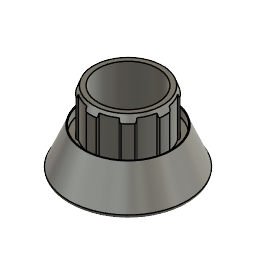
Fuß Tisch Keller (Autodesk Fusion 360 design; units mm, degrees)
Autodesk Fusion 360 part; units mm, degrees
sketch "Skizze1" plane through (0, 0, 0) normal (1, 0, 0) x (0, 0, -1)
  line L0 (0, 0) -> (-24, 0)
  line L1 (-24.9209, 1.3899) -> (-18.1, 17.5)
  line L2 (-18.1, 17.5) -> (-18.1, 13)
  line L3 (-18.1, 13) -> (-15, 13)
  line L4 (-15, 13) -> (-15, 31)
  line L5 (-15, 31) -> (-12.5, 31)
  line L6 (-12.5, 31) -> (-12.5, 4)
  arc A0 (-12.5, 4) -> (-11.5, 3) centre (-11.5, 4) ccw
  line L7 (-11.5, 3) -> (0, 3)
  line L8 (0, 3) -> (0, 0)
  arc A1 (-24.9209, 1.3899) -> (-24, 0) centre (-24, 1) ccw
  point P0 (-25.5093, 0)
  dimension "d1" = 31
  dimension "d2" = 18
  dimension "d3" = 12.5
  dimension "d4" = 3.1
  dimension "d5" = 15
  dimension "d6" = 13.5
  dimension "d7" = 1
  dimension "d8" = 28
  dimension "d28" = 1
  dimension "d29" = 24
  constraint coincident L0.start L8.end
  constraint horizontal L0
  constraint vertical L2
  constraint perpendicular L2 L3
  constraint perpendicular L3 L4
  constraint perpendicular L2 L5
  constraint perpendicular L5 L6
  constraint tangent L6 A0
  constraint tangent A0 L7
  constraint perpendicular L6 L7
  constraint perpendicular L0 L8
  constraint coincident P0 L0
  constraint coincident P0 L1
  constraint tangent L0 A1
  constraint tangent L1 A1
  measures "d1" vertical distance of L0.start L4.end
  measures "d2" distance of L3.end L4.end
  measures "d3" horizontal distance of L0.start L5.end
  measures "d4" distance of L2.end L3.end
  measures "d5" horizontal distance of L0.start L4.end
  measures "d6" vertical distance of L1.end L4.end
  measures "d7" radius of A0
  measures "d8" vertical distance of L5.end L7.end
  measures "d28" radius of A1
  measures "d29" horizontal distance of L0.start A1.centre
revolve "Drehen1" add sketch "Skizze1" angle 360 about axis through (0, 1.75, 0) along (0, 1, 0)
fillet "Abrundung1" radius 0.2 1 edges at (-16.8751, 17.5, 6.5452)
ref_plane "Arbeitsebene1" through (0, 30, 0) normal (0, 1, 0) x (0, 0, 1)
sketch "Skizze2" plane through (0, 30, 0) normal (0, 1, 0) x (1, 0, 0)
  arc A0 (-2.5929, -14.7742) -> (2.5929, -14.7742) centre (0, 0) ccw
  arc A1 (-2.08, -15.4607) -> (2.08, -15.4607) centre (0, 0) ccw
  arc A2 (2.08, -15.4607) -> (2.5929, -14.7742) centre (2, -14.8661) ccw
  arc A3 (-2.5929, -14.7742) -> (-2.08, -15.4607) centre (-2, -14.8661) ccw
  dimension "d15" = 15
  dimension "d16" = 15.6
  dimension "d30" = 4
  dimension "d31" = 2
  constraint coincident A0.centre A1.centre
  constraint tangent A1 A2
  constraint coincident A0.end A2.end
  constraint coincident A0 A2.centre
  constraint tangent A1 A3
  constraint coincident A0 A3.centre
  measures "d15" radius of A0
  measures "d16" radius of A1
  measures "d30" horizontal distance of A2.centre A3.centre
  measures "d31" horizontal distance of A0.centre A3.centre
extrude "Extrusion1" add sketch "Skizze2" against normal blind 18
sketch "Skizze3" plane through (0, 0, 0) normal (1, 0, 0) x (0, 0, -1)
  line L0 (-14.5, 31) -> (-15.6, 27.9778)
  line L1 (-15.6, 27.9778) -> (-15.6, 31)
  line L2 (-15.6, 31) -> (-14.5, 31)
  dimension "d21" = 14.5
  dimension "d22" = 1.1
  dimension "d23" = 20
  dimension "d24" = 31
  constraint vertical L1
  constraint perpendicular L1 L2
  measures "d21" horizontal distance of origin L0.start
  measures "d22" distance of L0.start L1.end
  measures "d23" angle of L0 L1
  measures "d24" vertical distance of origin L0.start
revolve "Drehen2" cut sketch "Skizze3" angle 360 about axis through (0, 1.75, 0) along (0, 1, 0)
pattern_circular "C-Anordnung1" count 8 over 360 about axis through (0, 1.75, 0) along (0, 1, 0) of "Extrusion1", "Drehen2"
